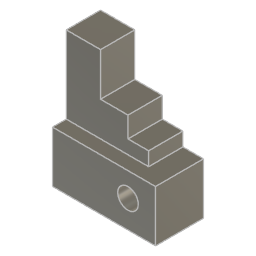
Practice problem 1 (Solid works) (Autodesk Fusion 360 design; units mm, degrees)
Autodesk Fusion 360 part; units mm, degrees
sketch "Sketch1" plane through (0, 0, 0) normal (0, 1, 0) x (1, 0, 0)
  line L0 (0, 0) -> (60, 0) construction
  line L1 (60, 0) -> (60, -30) construction
  line L2 (60, -30) -> (0, -30) construction
  line L3 (0, -30) -> (0, 0) construction
  line L4 (0, 0) -> (20, 0) construction
  line L5 (20, 0) -> (20, -75) construction
  line L6 (20, -75) -> (0, -75) construction
  line L7 (0, -75) -> (0, 0) construction
  line L8 (20, 0) -> (36, 0) construction
  line L9 (36, 0) -> (36, -75) construction
  line L10 (36, -75) -> (20, -75) construction
  line L11 (20, -75) -> (20, 0) construction
  line L12 (36, 0) -> (48, 0) construction
  line L13 (48, 0) -> (48, -75) construction
  line L14 (48, -75) -> (36, -75) construction
  line L15 (36, -75) -> (36, 0) construction
  line L16 (48, 0) -> (60, 0) construction
  line L17 (60, 0) -> (60, -75) construction
  line L18 (60, -75) -> (48, -75) construction
  line L19 (48, -75) -> (48, 0) construction
  line L20 (0, -75) -> (0, 0)
  line L21 (0, 0) -> (60, 0)
  line L22 (60, 0) -> (60, -30)
  line L23 (60, -30) -> (48, -30)
  line L24 (48, -30) -> (48, -38)
  line L25 (48, -38) -> (36, -38)
  line L26 (36, -38) -> (36, -50)
  line L27 (36, -50) -> (20, -50)
  line L28 (20, -50) -> (20, -75)
  line L29 (20, -75) -> (0, -75)
  line L30 (60, 0) -> (44, 0) construction
  line L31 (44, 0) -> (44, -30) construction
  line L32 (44, -30) -> (60, -30) construction
  line L33 (60, -30) -> (60, 0) construction
  line L34 (60, 0) -> (44, 0) construction
  line L35 (44, 0) -> (44, -16) construction
  line L36 (44, -16) -> (60, -16) construction
  line L37 (60, -16) -> (60, 0) construction
  circle A0 centre (44, -16) radius 6
  dimension "d1" = 60
  dimension "d2" = 30
  dimension "d3" = 75
  dimension "d4" = 16
  dimension "d5" = 12
  dimension "d6" = 12
  dimension "d7" = 16
  dimension "d8" = 20
  dimension "d9" = 25
  dimension "d10" = 16
  dimension "d11" = 16
  dimension "d12" = 12
  constraint horizontal L0
  constraint vertical L1
  constraint horizontal L2
  constraint vertical L3
  constraint coincident L0.start L3.end
  constraint horizontal L4
  constraint vertical L5
  constraint horizontal L6
  constraint vertical L7
  constraint horizontal L8
  constraint vertical L9
  constraint horizontal L10
  constraint vertical L11
  constraint horizontal L12
  constraint vertical L13
  constraint horizontal L14
  constraint vertical L15
  constraint horizontal L16
  constraint vertical L17
  constraint horizontal L18
  constraint vertical L19
  constraint coincident L13 L23.end
  constraint coincident L2 L23.end
  constraint coincident L19 L24.end
  constraint perpendicular L24 L25
  constraint perpendicular L25 L26
  constraint perpendicular L5 L27
  constraint perpendicular L20 L29
  constraint perpendicular L27 L28
  constraint horizontal L30
  constraint vertical L31
  constraint horizontal L32
  constraint vertical L33
  constraint coincident L0.end L1.start
  constraint horizontal L34
  constraint vertical L35
  constraint horizontal L36
  constraint vertical L37
  constraint coincident L35.end L36.start
  measures "d1" distance of L0.start L0.end
  measures "d2" distance of L0.start L2.end
  measures "d3" distance of L0.start L6.end
  measures "d4" distance of L4.end L8.end
  measures "d5" distance of L8.end L12.end
  measures "d6" distance of L25.end L26.end
  measures "d7" distance of L26.end L27.end
  measures "d8" distance of L6.end L5.end
  measures "d9" distance of L5.end L27.end
  measures "d10" distance of L0.end L30.end
  measures "d11" distance of L0.end L36.end
  measures "d12" diameter of A0
extrude "Extrude1" add sketch "Sketch1" along normal blind 28
sketch "Sketch2" plane through (0, 0, 0) normal (0, -1, 0) x (1, 0, 0)
  circle A0 centre (44, 16) radius 6
  line L0 (20, 50) -> (20, 75)
  line L1 (20, 75) -> (0, 75)
  line L2 (0, 75) -> (0, 0)
  line L3 (0, 0) -> (60, 0)
  line L4 (60, 0) -> (60, 30)
  line L5 (60, 30) -> (48, 30)
  line L6 (48, 30) -> (48, 38)
  line L7 (48, 38) -> (36, 38)
  line L8 (36, 38) -> (36, 50)
  line L9 (36, 50) -> (20, 50)
  line L10 (0, 0) -> (60, 0)
  line L11 (60, 0) -> (60, 30)
  line L12 (60, 30) -> (0, 30)
  line L13 (0, 30) -> (0, 0)
  constraint horizontal L10
  constraint vertical L11
  constraint horizontal L12
  constraint vertical L13
  constraint coincident L4.end L5.start
  constraint coincident L2.end L3.start
extrude "Extrude2" cut sketch "Sketch2" against normal blind 8 contours L0 L1 L2 L6 L7 L8 L9 L12
